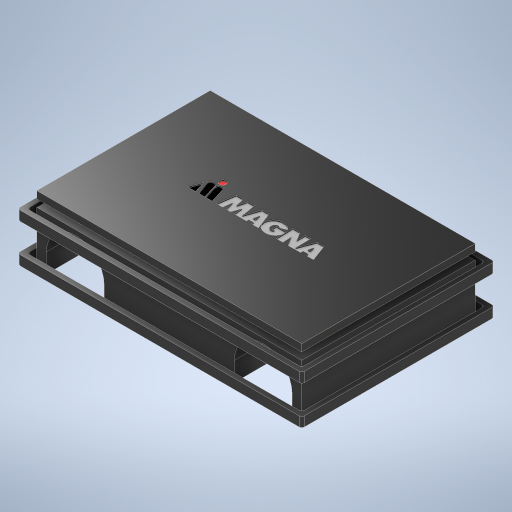
# Autodesk Inventor part: platform
Saved by Autodesk Inventor 2024 (Build 280153000, 153)
## iProperties
Created: 2024-04-03
Part Number: platform
Material: Generic
Document SubType Name: Modeling
Designer: Gabek
Density: 1 g/cm^3
Appearance: Glossy - Black
Author: Gabek
Autodesk Inventor part; units mm, degrees
ref_plane "YZ Plane" through (0, 0, 0) normal (1, 0, 0) x (0, 1, 0)
ref_plane "XZ Plane" through (0, 0, 0) normal (0, 1, 0) x (-1, 0, 0)
ref_plane "XY Plane" through (0, 0, 0) normal (0, 0, 1) x (1, 0, 0)
sketch "Sketch1" plane through (0, 0, 0) normal (0, 1, 0) x (-1, 0, 0)
  line L0 (-698.5, -457.2) -> (698.5, -457.2)
  line L1 (698.5, -457.2) -> (698.5, 457.2)
  line L2 (698.5, 457.2) -> (-698.5, 457.2)
  line L3 (-698.5, 457.2) -> (-698.5, -457.2)
  line L4 (-698.5, -457.2) -> (698.5, 457.2) construction
  line L5 (698.5, -457.2) -> (-698.5, 457.2) construction
  point P0 (0, 0)
  dimension "d0" = 914.4
  dimension "d1" = 1397
  constraints: 12 end point, 2 midpoint, 2 parallel, 1 horizontal, 1 perpendicular
  measures "d0" distance of L0.end L1.end
  measures "d1" distance of L1.end L2.end
extrude "Extrusion1" add sketch "Sketch1" along normal blind 355.6
sketch "Sketch2" plane through (-698.5, 0, 457.2) normal (0, 0, 1) x (1, 0, 0)
  arc A0 (1346.2, 101.6) -> (1041.4, 101.6) centre (1193.8, 101.6) ccw
  line L0 (0, 0) -> (1397, 0) projected
  line L1 (1397, 0) -> (1397, 355.6) projected
  line L2 (1346.2, 101.6) -> (1346.2, 0)
  line L3 (1041.4, 101.6) -> (1041.4, 0)
  line L4 (1041.4, 0) -> (1346.2, 0)
  line L5 (1307.3923, 0) -> (1346.2, 0)
  point P0 (698.5, 0)
  dimension "d4" = 101.6
  dimension "d5" = 304.8
  dimension "d6" = 203.2
  constraints: 8 end point, 2 collinear, 2 perpendicular, 2 point on circle, 2 point on line, 2 tangent, 1 centre point
  measures "d4" distance from line of L0 A0.centre
  measures "d5" diameter of A0
  measures "d6" distance from line of L1 A0.centre
extrude "Extrusion2" cut sketch "Sketch2" against normal blind 203.2
mirror "Mirror1" about plane through (0, 0, 0) normal (0, 0, 1) of "Extrusion2"
mirror "Mirror2" about plane through (0, 0, 0) normal (1, 0, 0) of "Extrusion2", "Mirror1"
sketch "Sketch3" plane through (-698.5, 355.6, 457.2) normal (0, 0, 1) x (1, 0, 0)
  line L0 (0, -355.6) -> (0, 0) projected
  line L1 (0, -38.1) -> (38.1, -38.1)
  line L2 (38.1, -38.1) -> (38.1, -76.2)
  line L3 (38.1, -76.2) -> (0, -76.2)
  line L4 (0, -76.2) -> (0, -38.1)
  line L5 (0, 0) -> (1397, 0) projected
  point P0 (698.5, -355.6)
  point P1 (0, -76.2)
  dimension "d9" = 38.1
  dimension "d10" = 38.1
  dimension "d11" = 38.1
  constraints: 8 end point, 2 parallel, 1 horizontal, 1 perpendicular, 1 point on line
  measures "d9" distance of L1.start L1.end
  measures "d10" distance of L1.end L2.end
  measures "d11" distance between parallel lines of L5 L1
sketch3d "3D Sketch1"
  line L0 (-698.5, 355.6, 457.2) -> (-698.5, 355.6, -457.2)
  line L1 (-698.5, 355.6, -457.2) -> (698.5, 355.6, -457.2)
  line L2 (698.5, 355.6, -457.2) -> (698.5, 355.6, 457.2)
  line L3 (698.5, 355.6, 457.2) -> (-698.5, 355.6, 457.2)
sweep "Sweep1" cut profiles "Sketch3" path "3D Sketch1"
sketch "Sketch4" plane through (647.7, 0, 457.2) normal (0, 0, 1) x (1, 0, 0)
  line L0 (-914.4, 44.45) -> (-381, 44.45)
  line L1 (-381, 44.45) -> (-381, 19.05)
  line L2 (-381, 19.05) -> (-914.4, 19.05)
  line L3 (-914.4, 19.05) -> (-914.4, 44.45)
  line L4 (-990.6, 101.6) -> (-990.6, 0) projected
  line L5 (-304.8, 0) -> (-304.8, 101.6) projected
  line L6 (-990.6, 0) -> (-304.8, 0) projected
  point P0 (-647.7, 0)
  dimension "d14" = 76.2
  dimension "d15" = 76.2
  dimension "d16" = 25.4
  dimension "d17" = 19.05
  constraints: 8 end point, 2 parallel, 1 horizontal, 1 perpendicular
  measures "d14" distance between parallel lines of L4 L3
  measures "d15" distance between parallel lines of L5 L1
  measures "d16" distance of L2.end L0.start
  measures "d17" distance between parallel lines of L6 L2
extrude "Extrusion3" add sketch "Sketch4" along normal blind 25.4
sketch "Sketch5" plane through (-266.7, 19.05, 457.2) normal (-1, 0, 0) x (0, 0, 1)
  line L0 (25.4, 0) -> (50.8, 0)
  line L1 (50.8, 0) -> (50.8, 50.8)
  line L2 (50.8, 50.8) -> (25.4, 50.8)
  line L3 (25.4, 50.8) -> (25.4, 0)
  point P0 (-457.2, -19.05)
  dimension "d20" = 50.8
  constraints: 8 end point, 2 parallel, 1 horizontal, 1 perpendicular
  measures "d20" distance of L1.end L0.end
sketch3d "3D Sketch2"
  line L0 (-698.5, 355.6, 457.2) -> (698.5, 355.6, 457.2)
  line L1 (698.5, 355.6, 457.2) -> (698.5, 355.6, -457.2)
  line L2 (698.5, 355.6, -457.2) -> (-698.5, 355.6, -457.2)
  line L3 (-698.5, 355.6, -457.2) -> (-698.5, 355.6, 457.2)
sweep "Sweep2" add profiles "Sketch5" path "3D Sketch2"
mirror "Mirror3" about plane through (0, 0, 0) normal (0, 0, 1) of "Extrusion3"
sketch "Sketch6" plane through (698.5, 0, 457.2) normal (1, 0, 0) x (0, 0, -1)
  line L0 (939.8, 19.05) -> (-25.4, 19.05) projected
  line L1 (101.6, 44.45) -> (304.8, 44.45)
  line L2 (304.8, 44.45) -> (304.8, 19.05)
  line L3 (304.8, 19.05) -> (101.6, 19.05)
  line L4 (101.6, 19.05) -> (101.6, 44.45)
  line L5 (609.6, 44.45) -> (812.8, 44.45)
  line L6 (812.8, 44.45) -> (812.8, 19.05)
  line L7 (812.8, 19.05) -> (609.6, 19.05)
  line L8 (609.6, 19.05) -> (609.6, 44.45)
  line L9 (0, 101.6) -> (0, 0) projected
  line L10 (914.4, 0) -> (914.4, 101.6) projected
  point P0 (457.2, 0)
  point P1 (304.8, 31.75)
  point P2 (609.6, 31.75)
  point P3 (101.6, 31.75)
  point P4 (101.6, 19.05)
  dimension "d23" = 152.4
  dimension "d24" = 152.4
  dimension "d25" = 25.4
  dimension "d26" = 25.4
  dimension "d27" = 101.6
  dimension "d28" = 101.6
  constraints: 16 end point, 4 parallel, 3 midpoint, 2 horizontal, 2 perpendicular, 2 point on line
  measures "d23" horizontal distance of point (457.2, 0) point (304.8, 31.75)
  measures "d24" horizontal distance of point (609.6, 31.75) point (457.2, 0)
  measures "d25" distance between parallel lines of L0 L5
  measures "d26" distance between parallel lines of L0 L1
  measures "d27" distance from line of L9 point (101.6, 31.75)
  measures "d28" distance from line of L10 L6.end
extrude "Extrusion4" add sketch "Sketch6" along normal blind 25.4
mirror "Mirror4" about plane through (0, 0, 0) normal (1, 0, 0) of "Extrusion4"
fillet "Fillet1" radius 12.7 8 edges at (749.3, 44.45, -508) (-749.3, 44.45, -508) (-723.9, 44.45, -482.6) (-723.9, 44.45, 482.6) (-749.3, 44.45, 508) (723.9, 44.45, 482.6) (749.3, 44.45, 508) (723.9, 44.45, -482.6)
pattern_linear "Rectangular Pattern1" count 2 spacing 203.2 along (0, 1, 0) of "Fillet1", "Extrusion4", "Mirror4", "Extrusion3", "Sweep2", "Mirror3"
sketch "Sketch7" plane through (698.5, 0, -457.2) normal (0, 0, -1) x (-1, 0, 0)
  line L0 (-12.7, 273.05) -> (1409.7, 273.05) projected
  line L1 (1435.1, 19.05) -> (-38.1, 19.05) projected
  line L2 (431.8, 273.05) -> (965.2, 273.05)
  line L3 (965.2, 273.05) -> (965.2, 19.05)
  line L4 (965.2, 19.05) -> (431.8, 19.05)
  line L5 (431.8, 19.05) -> (431.8, 273.05)
  line L6 (431.8, 222.25) -> (431.8, 247.65) projected
  line L7 (965.2, 247.65) -> (965.2, 222.25) projected
  point P0 (698.5, 0)
  point P1 (431.8, 19.05)
  constraints: 8 end point, 2 collinear, 2 parallel, 2 point on line, 1 horizontal, 1 perpendicular
extrude "Extrusion5" add sketch "Sketch7" along normal blind 50.8
sketch "Sketch8" plane through (-495.3, 101.6, 254) normal (0, 0, 1) x (1, 0, 0)
  circle A0 centre (0, 0) radius 6.35
  point P0 (495.3, -101.6)
  dimension "d37" = 12.7
  constraints: 1 centre point
  measures "d37" diameter of A0
extrude "Extrusion6" add sketch "Sketch8" along normal blind 50.8
mirror "Mirror5" about plane through (0, 0, 0) normal (1, 0, 0) of "Extrusion6"
mirror "Mirror6" about plane through (0, 0, 0) normal (0, 0, 1) of "Extrusion6", "Mirror5"
sketch "Sketch9" plane through (0, 355.6, 0) normal (0, 1, 0) x (1, 0, 0)
  line L0 (-377.343, 395.3194) -> (398.9445, 395.3194) construction
  line L1 (398.9445, 395.3194) -> (398.9445, -380.9681) construction
  line L2 (398.9445, -380.9681) -> (-377.343, -380.9681) construction
  line L3 (-377.343, -380.9681) -> (-377.343, 395.3194) construction
  line L4 (-282.1677, 47.7027) -> (-255.1802, 47.7027)
  line L5 (-255.1802, 47.7027) -> (-227.5501, -42.8625)
  line L6 (-227.5501, -42.8625) -> (-260.35, -42.8625)
  line L7 (-260.35, -42.8625) -> (-289.1691, 32.6802)
  line L8 (-289.1691, 32.6802) -> (-282.1677, 47.7027)
  line L9 (-295.275, 19.5792) -> (-319.0875, -42.8625)
  line L10 (-319.0875, -42.8625) -> (-276.225, -42.8625)
  line L11 (-276.225, -42.8625) -> (-295.275, 19.5792)
  line L12 (-242.8673, 47.7027) -> (-247.7018, 35.0256)
  line L13 (-247.7018, 35.0256) -> (-223.9394, -42.8625)
  line L14 (-223.9394, -42.8625) -> (-188.4045, -42.8625)
  line L15 (-188.4045, -42.8625) -> (-216.0345, 47.7027)
  line L16 (-216.0345, 47.7027) -> (-242.8673, 47.7027)
  line L17 (-165.1, -42.8625) -> (-151.9038, 47.7027)
  line L18 (-151.9038, 47.7027) -> (-115.8875, 47.7027)
  line L19 (-115.8875, 47.7027) -> (-103.3657, 0)
  line L20 (-103.3657, 0) -> (-91.2323, 47.7027)
  line L21 (-91.2323, 47.7027) -> (-56.373, 47.7027)
  line L22 (-56.373, 47.7027) -> (-42.8625, -30.2596)
  line L23 (-42.8625, -30.2596) -> (-15.875, 47.7027)
  line L24 (-15.875, 47.7027) -> (20.6276, 47.7027)
  line L25 (20.6276, 47.7027) -> (55.5625, -42.8625)
  line L26 (55.5625, -42.8625) -> (19.05, -42.8625)
  line L27 (19.05, -42.8625) -> (19.05, -30.2596)
  line L28 (19.05, -30.2596) -> (-7.9375, -30.2596)
  line L29 (-7.9375, -30.2596) -> (-7.9375, -42.8625)
  line L30 (-7.9375, -42.8625) -> (-71.4375, -42.8625)
  line L31 (-71.4375, -42.8625) -> (-75.5131, 2.4201)
  line L32 (-75.5131, 2.4201) -> (-92.1144, -42.8625)
  line L33 (-92.1144, -42.8625) -> (-112.7125, -42.8625)
  line L34 (-112.7125, -42.8625) -> (-127.6756, 6.1833)
  line L35 (-127.6756, 6.1833) -> (-133.8956, -42.8625)
  line L36 (-133.8956, -42.8625) -> (-165.1, -42.8625)
  line L37 (11.1125, -12.6081) -> (-3.175, -12.6081)
  line L38 (-3.175, -12.6081) -> (4.4735, 17.4625)
  line L39 (4.4735, 17.4625) -> (11.1125, -12.6081)
  line L40 (141.4022, 24.8319) -> (114.3, 14.3774)
  line L41 (149.066, 45.9001) -> (185.7375, 45.9001)
  line L42 (185.7375, 45.9001) -> (214.3125, 0)
  line L43 (214.3125, 0) -> (214.3125, 45.9001)
  line L44 (214.3125, 45.9001) -> (242.8875, 45.9001)
  line L45 (242.8875, 45.9001) -> (244.475, -36.5611)
  line L46 (244.475, -36.5611) -> (276.1196, 45.9001)
  line L47 (276.1196, 45.9001) -> (312.7307, 46.6049)
  line L48 (312.7307, 46.6049) -> (346.075, -42.8625)
  line L49 (346.075, -42.8625) -> (311.15, -43.5349)
  line L50 (311.15, -43.5349) -> (306.2023, -30.2596)
  line L51 (306.2023, -30.2596) -> (279.4, -30.2596)
  line L52 (279.4, -30.2596) -> (279.4, -44.1461)
  line L53 (279.4, -44.1461) -> (214.3125, -45.3991)
  line L54 (214.3125, -45.3991) -> (183.1424, 4.6695)
  line L55 (183.1424, 4.6695) -> (185.7375, -44.1461)
  line L56 (185.7375, -44.1461) -> (150.8125, -44.8185)
  line L57 (150.8125, -44.8185) -> (149.0525, 46.6049)
  line L58 (292.8012, 17.4625) -> (285.75, -12.6081)
  line L59 (285.75, -12.6081) -> (299.6237, -12.6081)
  line L60 (299.6237, -12.6081) -> (292.0778, 14.3774)
  ellipse E0 centre (96.8211, -0.1293) end of major axis (44.4228, -0.1293) minor radius 47.5028 (141.4022, 24.8319) -> (147.6333, 11.4695) ccw
  ellipse E1 centre (96.8211, -0.1293) end of major axis (96.8211, 20.1014) minor radius 17.4461 (108.9811, 14.3774) -> (110.5528, -12.6081) ccw
  line L61 (110.5528, -12.6081) -> (96.935, -12.6081)
  line L62 (96.935, -12.6081) -> (96.935, 11.4695)
  line L63 (96.935, 11.4695) -> (147.6333, 11.4695)
  line L64 (114.3, 14.3774) -> (108.9811, 14.3774)
  circle A0 centre (-245.2846, 69.85) radius 17.1377
  point P0 (0, 0)
  constraints: 122 end point, 30 point on line, 13 parallel, 10 perpendicular, 7 horizontal, 1 centre point, 1 coincident, 1 collinear, 10 other
extrude "Extrusion7" cut sketch "Sketch9" against normal blind 6.35
body "Solid1"
